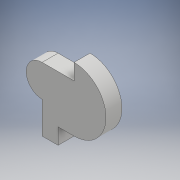
# Autodesk Inventor part: 44
Saved by Autodesk Inventor 2017 (Build 210142000, 142)
## iProperties
Part Number: 44
Material: 一般
Document SubType Name: Modeling
Designer: Brian
Density: 1 g/cm^3
Appearance: 預設
Author: Brian
Autodesk Inventor part; units mm, degrees
ref_plane "YZ Plane" through (0, 0, 0) normal (1, 0, 0) x (0, 1, 0)
ref_plane "XZ Plane" through (0, 0, 0) normal (0, 1, 0) x (-1, 0, 0)
ref_plane "XY Plane" through (0, 0, 0) normal (0, 0, 1) x (1, 0, 0)
sketch "草圖1" plane through (0, 0, 0) normal (0, 1, 0) x (-1, 0, 0)
  line L0 (0, 0) -> (-20, 0)
  line L1 (-20, 0) -> (-20, -20)
  line L2 (-20, -20) -> (0, -20)
  line L3 (0, -20) -> (0, 0)
  line L4 (-20, 0) -> (-30, 0)
  line L5 (-30, 0) -> (-30, -30)
  line L6 (-30, -30) -> (-20, -30)
  line L7 (-20, -30) -> (-20, 0)
  line L8 (-30, -30) -> (-50, -30)
  line L9 (-50, -30) -> (-50, 10)
  line L10 (-50, 10) -> (-30, 10)
  line L11 (-30, 10) -> (-30, -30)
  dimension "d0" = 20
  dimension "d1" = 20
  dimension "d2" = 20
  dimension "d3" = 10
  dimension "d4" = 30
  dimension "d5" = 40
  constraints: 24 end point, 6 parallel, 3 horizontal, 3 perpendicular
  measures "d0" distance of L5.end L8.end
  measures "d1" distance of L1.end L2.end
  measures "d2" distance of L2.end L0.start
  measures "d3" distance of L5.end L6.end
  measures "d4" distance of L6.end L0.end
  measures "d5" distance of L8.end L9.end
extrude "擠出1" add sketch "草圖1" along normal blind 10
fillet "圓角1" radius 20 2 edges at (50, 5, 10) (50, 5, -30)
fillet "圓角2" radius 10 2 edges at (0, 5, -20) (0, 5, 0)
sketch "草圖2" plane through (20, 0, -30) normal (-1, 0, 0) x (0, 0, 1)
  line L0 (10, 0) -> (10, 10) projected
  line L1 (10, 10) -> (-10, 30)
  line L2 (-10, 30) -> (-10, 0)
  line L3 (-10, 0) -> (10, 0)
  point P0 (30, 0)
  dimension "d10" = 20
  dimension "d11" = 30
  constraints: 6 end point, 1 parallel, 1 perpendicular
  measures "d10" distance of L2.end L0.start
  measures "d11" distance of L1.end L2.end
extrude "擠出2" add sketch "草圖2" along normal blind 10
